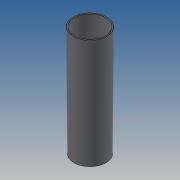
# Autodesk Inventor part: FLY MEDIA TUBE
Saved by Autodesk Inventor 2018.3 (Build 223284000, 284)
## iProperties
Created: 2018-09-09
Material: Generic
Vendor: HHMI: JRC - ID&F
Document SubType Name: Modeling
Designer: arnoldj
Density: 1 g/cm^3
Appearance: Default
RuleStatus: InUse
AfterDocSave0: file://Part Number Cleaner
DESIGN DEPARTMENT: HHMI: JRC - ID&F
ALTERED ITEM PART NUMBER: N/A
ALTERED ITEM VENDOR: N/A
ALTERED ITEM DESCRIPTION: N/A
Author: arnoldj
Revision Number: 0
Autodesk Inventor part; units mm, degrees
ref_plane "YZ Plane" through (0, 0, 0) normal (1, 0, 0) x (0, 1, 0)
ref_plane "XZ Plane" through (0, 0, 0) normal (0, 1, 0) x (-1, 0, 0)
ref_plane "XY Plane" through (0, 0, 0) normal (0, 0, 1) x (1, 0, 0)
sketch "Sketch1" plane through (0, 0, 0) normal (0, 0, 1) x (1, 0, 0)
  line L0 (0, 116.9344) -> (0, -19.4891) projected
  line L1 (-17.2212, 0) -> (2.8702, 0) projected
  line L2 (0, 0) -> (0, 97.4453)
  line L3 (0, 0) -> (-13.6144, 0)
  line L4 (-13.6144, 0) -> (-14.351, 93.9546)
  line L5 (-14.351, 93.9546) -> (-13.2588, 93.9546)
  line L6 (-13.2588, 93.9546) -> (-12.5373, 1.9304)
  line L7 (-12.5373, 0) -> (-12.5373, 0.8382)
  line L8 (-12.5373, 0.8382) -> (0, 0.8382)
  line L9 (-12.5373, 1.9304) -> (0, 1.9304)
  line L10 (0, 1.9304) -> (0, 0.8382)
  dimension "d0" = 27.2288
  dimension "d1" = 28.702
  dimension "d2" = 93.9546
  dimension "d3" = 1.0922
  dimension "d5" = 0.8382
  dimension "d6" = 1.0922
  dimension "d9" = 26.5175
  constraints: 18 end point, 4 point on line, 3 perpendicular, 1 collinear, 1 parallel, 1 vertical, 1 vertical alignment
  measures "d0" diameter of L3.end L2
  measures "d1" diameter of L4.end L2
  measures "d2" distance between parallel lines of L1 L5
  measures "d3" distance between parallel lines of L4 L6
  measures "d5" distance between parallel lines of L8 L1
  measures "d6" distance between parallel lines of L9 L8
  measures "d9" diameter of L5.end L2
revolve "Revolution1" add sketch "Sketch1" angle 360 about axis through (0, 0, 0) along (0, 1, 0) contours L0 L8 L7 L1 L4 L5 L6 L9
fillet "Fillet1" radius 0.254 2 edges at (13.2588, 93.9546, 0) (14.351, 93.9546, 0)
body "Solid1"
